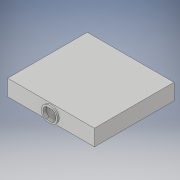
# Autodesk Inventor part: room with 15 cubicals
Saved by Autodesk Inventor 2017 (Build 210142000, 142)
## iProperties
Created: 2018-03-22
Part Number: room with 15 cubicals
Material: Generic
Document SubType Name: Modeling
Designer: Braxton
Density: 1 g/cm^3
Appearance: Default
Author: Braxton
Autodesk Inventor part; units mm, degrees
ref_plane "YZ Plane" through (0, 0, 0) normal (1, 0, 0) x (0, 1, 0)
ref_plane "XZ Plane" through (0, 0, 0) normal (0, 1, 0) x (-1, 0, 0)
ref_plane "XY Plane" through (0, 0, 0) normal (0, 0, 1) x (1, 0, 0)
sketch "Sketch1" plane through (0, 0, 0) normal (0, 1, 0) x (-1, 0, 0)
  line L0 (0, 0) -> (0, -304.8)
  line L1 (0, -304.8) -> (-203.2, -304.8)
  line L2 (-203.2, -304.8) -> (-203.2, -63.5)
  line L3 (0, 0) -> (-203.2, 0)
  line L4 (-205.3167, -63.5) -> (-205.3167, -306.9167)
  line L5 (2.1167, -306.9167) -> (2.1167, 2.1167)
  line L6 (2.1167, 2.1167) -> (-203.2, 2.1167)
  line L7 (-203.2, -63.5) -> (-205.3167, -63.5)
  line L8 (-203.2, 0) -> (-205.3167, 0)
  line L9 (-205.3167, 0) -> (-205.3167, 2.1167)
  line L10 (-205.3167, 2.1167) -> (-203.2, 2.1167)
  line L11 (0, -304.8) -> (-203.2, -304.8)
  line L12 (-281.5167, -920.75) -> (-281.5167, 2.1167) construction
  line L13 (0, -306.9167) -> (-205.3167, -306.9167)
  line L14 (0, -306.9167) -> (0, -611.7167)
  line L15 (0, -611.7167) -> (-203.2, -611.7167)
  line L16 (-203.2, -611.7167) -> (-203.2, -370.4167)
  line L17 (-205.3167, -370.4167) -> (-205.3167, -613.8333)
  line L18 (2.1167, -613.8333) -> (2.1167, -306.9167)
  line L19 (-203.2, -370.4167) -> (-205.3167, -370.4167)
  line L20 (0, -611.7167) -> (-203.2, -611.7167)
  line L21 (0, -613.8333) -> (-205.3167, -613.8333)
  line L22 (0, -613.8333) -> (0, -918.6333)
  line L23 (0, -918.6333) -> (-203.2, -918.6333)
  line L24 (-203.2, -918.6333) -> (-203.2, -677.3333)
  line L25 (-205.3167, -677.3333) -> (-205.3167, -920.75)
  line L26 (2.1167, -920.75) -> (2.1167, -613.8333)
  line L27 (-203.2, -677.3333) -> (-205.3167, -677.3333)
  line L28 (0, -918.6333) -> (-203.2, -918.6333)
  line L29 (2.1167, -920.75) -> (-205.3167, -920.75)
  line L30 (-563.0333, 0) -> (-563.0333, -304.8)
  line L31 (-563.0333, -304.8) -> (-359.8333, -304.8)
  line L32 (-359.8333, -304.8) -> (-359.8333, -63.5)
  line L33 (-563.0333, 0) -> (-359.8333, 0)
  line L34 (-357.7167, -63.5) -> (-357.7167, -306.9167)
  line L35 (-565.15, -306.9167) -> (-565.15, 2.1167)
  line L36 (-565.15, 2.1167) -> (-359.8333, 2.1167)
  line L37 (-359.8333, -63.5) -> (-357.7167, -63.5)
  line L38 (-359.8333, 0) -> (-357.7167, 0)
  line L39 (-357.7167, 0) -> (-357.7167, 2.1167)
  line L40 (-357.7167, 2.1167) -> (-359.8333, 2.1167)
  line L41 (-563.0333, -304.8) -> (-359.8333, -304.8)
  line L42 (-563.0333, -306.9167) -> (-357.7167, -306.9167)
  line L43 (-563.0333, -613.8333) -> (-357.7167, -613.8333)
  line L44 (-563.0333, -611.7167) -> (-359.8333, -611.7167)
  line L45 (-563.0333, -611.7167) -> (-359.8333, -611.7167)
  line L46 (-357.7167, -370.4167) -> (-357.7167, -613.8333)
  line L47 (-359.8333, -611.7167) -> (-359.8333, -370.4167)
  line L48 (-359.8333, -370.4167) -> (-357.7167, -370.4167)
  line L49 (-563.0333, -306.9167) -> (-563.0333, -611.7167)
  line L50 (-565.15, -613.8333) -> (-565.15, -306.9167)
  line L51 (-565.15, -920.75) -> (-357.7167, -920.75)
  line L52 (-563.0333, -918.6333) -> (-359.8333, -918.6333)
  line L53 (-563.0333, -918.6333) -> (-359.8333, -918.6333)
  line L54 (-357.7167, -677.3333) -> (-357.7167, -920.75)
  line L55 (-359.8333, -918.6333) -> (-359.8333, -677.3333)
  line L56 (-359.8333, -677.3333) -> (-357.7167, -677.3333)
  line L57 (-563.0333, -613.8333) -> (-563.0333, -918.6333)
  line L58 (-565.15, -920.75) -> (-565.15, -613.8333)
  line L59 (-641.35, -920.75) -> (-641.35, 2.1167) construction
  line L60 (-1282.7, 0) -> (-1282.7, -304.8)
  line L61 (-1282.7, -304.8) -> (-1079.5, -304.8)
  line L62 (-1079.5, -304.8) -> (-1079.5, -63.5)
  line L63 (-1282.7, 0) -> (-1079.5, 0)
  line L64 (-1077.3833, -63.5) -> (-1077.3833, -306.9167)
  line L65 (-1284.8167, -306.9167) -> (-1284.8167, 2.1167)
  line L66 (-1284.8167, 2.1167) -> (-1079.5, 2.1167)
  line L67 (-1079.5, -63.5) -> (-1077.3833, -63.5)
  line L68 (-1079.5, 0) -> (-1077.3833, 0)
  line L69 (-1077.3833, 0) -> (-1077.3833, 2.1167)
  line L70 (-1077.3833, 2.1167) -> (-1079.5, 2.1167)
  line L71 (-1282.7, -304.8) -> (-1079.5, -304.8)
  line L72 (-1001.1833, -920.75) -> (-1001.1833, 2.1167) construction
  line L73 (-1282.7, -306.9167) -> (-1077.3833, -306.9167)
  line L74 (-1282.7, -613.8333) -> (-1077.3833, -613.8333)
  line L75 (-1282.7, -611.7167) -> (-1079.5, -611.7167)
  line L76 (-1282.7, -611.7167) -> (-1079.5, -611.7167)
  line L77 (-1077.3833, -370.4167) -> (-1077.3833, -613.8333)
  line L78 (-1079.5, -611.7167) -> (-1079.5, -370.4167)
  line L79 (-1079.5, -370.4167) -> (-1077.3833, -370.4167)
  line L80 (-1282.7, -306.9167) -> (-1282.7, -611.7167)
  line L81 (-1284.8167, -613.8333) -> (-1284.8167, -306.9167)
  line L82 (-1284.8167, -920.75) -> (-1077.3833, -920.75)
  line L83 (-1282.7, -918.6333) -> (-1079.5, -918.6333)
  line L84 (-1282.7, -918.6333) -> (-1079.5, -918.6333)
  line L85 (-1077.3833, -677.3333) -> (-1077.3833, -920.75)
  line L86 (-1079.5, -918.6333) -> (-1079.5, -677.3333)
  line L87 (-1079.5, -677.3333) -> (-1077.3833, -677.3333)
  line L88 (-1282.7, -613.8333) -> (-1282.7, -918.6333)
  line L89 (-1284.8167, -920.75) -> (-1284.8167, -613.8333)
  line L90 (-719.6667, 0) -> (-719.6667, -304.8)
  line L91 (-719.6667, -304.8) -> (-922.8667, -304.8)
  line L92 (-922.8667, -304.8) -> (-922.8667, -63.5)
  line L93 (-719.6667, 0) -> (-922.8667, 0)
  line L94 (-922.8667, -63.5) -> (-924.9833, -63.5)
  line L95 (-922.8667, 0) -> (-924.9833, 0)
  line L96 (-924.9833, 0) -> (-924.9833, 2.1167)
  line L97 (-924.9833, 2.1167) -> (-922.8667, 2.1167)
  line L98 (-717.55, -306.9167) -> (-717.55, 2.1167)
  line L99 (-717.55, 2.1167) -> (-922.8667, 2.1167)
  line L100 (-719.6667, -304.8) -> (-922.8667, -304.8)
  line L101 (-924.9833, -63.5) -> (-924.9833, -306.9167)
  line L102 (-719.6667, -306.9167) -> (-924.9833, -306.9167)
  line L103 (-922.8667, -370.4167) -> (-924.9833, -370.4167)
  line L104 (-719.6667, -306.9167) -> (-719.6667, -611.7167)
  line L105 (-717.55, -613.8333) -> (-717.55, -306.9167)
  line L106 (-719.6667, -611.7167) -> (-922.8667, -611.7167)
  line L107 (-719.6667, -611.7167) -> (-922.8667, -611.7167)
  line L108 (-719.6667, -613.8333) -> (-924.9833, -613.8333)
  line L109 (-924.9833, -370.4167) -> (-924.9833, -613.8333)
  line L110 (-922.8667, -611.7167) -> (-922.8667, -370.4167)
  line L111 (-922.8667, -918.6333) -> (-922.8667, -677.3333)
  line L112 (-924.9833, -677.3333) -> (-924.9833, -920.75)
  line L113 (-719.6667, -613.8333) -> (-719.6667, -918.6333)
  line L114 (-717.55, -920.75) -> (-717.55, -613.8333)
  line L115 (-719.6667, -918.6333) -> (-922.8667, -918.6333)
  line L116 (-719.6667, -918.6333) -> (-922.8667, -918.6333)
  line L117 (-717.55, -920.75) -> (-924.9833, -920.75)
  line L118 (-922.8667, -677.3333) -> (-924.9833, -677.3333)
  dimension "d4" = 304.8
  dimension "d5" = 203.2
  dimension "d7" = 63.5
  dimension "d95" = 2.1167
  dimension "d97" = 2.1167
  dimension "d98" = 2.1167
  dimension "d99" = 304.8
  dimension "d100" = 203.2
  dimension "d102" = 2.1167
  dimension "d103" = 2.1167
  dimension "d104" = 2.1167
  dimension "d106" = 304.8
  dimension "d107" = 203.2
  dimension "d109" = 2.1167
  dimension "d110" = 2.1167
  dimension "d111" = 2.1167
  dimension "d113" = 63.5
  dimension "d114" = 63.5
  dimension "d115" = 76.2
  dimension "d117" = 76.2
  constraints: 238 end point, 80 symmetric about line, 8 perpendicular, 8 vertical, 7 horizontal, 6 collinear, 4 point on line, 1 other
  measures "d4" distance of L0.end L0.start
  measures "d5" distance of L1.end L0.end
  measures "d7" distance from line of L3 L2.end
  measures "d95" distance between parallel lines of L0 L5
  measures "d97" distance between parallel lines of L1 L13
  measures "d98" distance between parallel lines of L2 L4
  measures "d99" distance of L15.start L13.start
  measures "d100" distance of L15.end L15.start
  measures "d102" distance between parallel lines of L14 L18
  measures "d103" distance between parallel lines of L15 L21
  measures "d104" distance between parallel lines of L16 L17
  measures "d106" distance of L23.start L21.start
  measures "d107" distance of L23.end L23.start
  measures "d109" distance between parallel lines of L22 L26
  measures "d110" distance between parallel lines of L23 L29
  measures "d111" distance between parallel lines of L24 L25
  measures "d113" distance between parallel lines of L13 L19
  measures "d114" distance between parallel lines of L21 L27
  measures "d115" distance between parallel lines of L25 L12
  measures "d117" distance between parallel lines of L59 L58
extrude "cubicals" add sketch "Sketch1" along normal blind 114.3
sketch "Sketch2" plane through (0, 0, 0) normal (0, -1, 0) x (1, 0, 0)
  line L0 (1310.2167, 154.5167) -> (-27.5167, 154.5167)
  line L1 (-27.5167, 154.5167) -> (-27.5167, -1073.15)
  line L2 (-27.5167, -1073.15) -> (1310.2167, -1073.15)
  line L3 (1310.2167, -1073.15) -> (1310.2167, 154.5167)
  line L4 (-2.1167, -920.75) -> (-2.1167, 2.1167) projected
  line L5 (1284.8167, 2.1167) -> (1284.8167, -920.75) projected
  line L6 (1284.8167, -920.75) -> (1077.3833, -920.75) projected
  line L7 (717.55, 2.1167) -> (924.9833, 2.1167) projected
  point P0 (0, 0)
  dimension "d118" = 152.4
  dimension "d120" = 152.4
  dimension "d128" = 25.4
  dimension "d129" = 25.4
  constraints: 8 end point, 2 parallel, 1 horizontal, 1 perpendicular
  measures "d118" distance between parallel lines of L6 L2
  measures "d120" distance between parallel lines of L0 L7
  measures "d128" distance between parallel lines of L1 L4
  measures "d129" distance between parallel lines of L3 L5
extrude "floor" add sketch "Sketch2" along normal blind 25.4
sketch "Sketch3" plane through (0, 0, 0) normal (0, 1, 0) x (1, 0, 0)
  line L0 (-27.5167, -154.5167) -> (-27.5167, 1073.15) projected
  line L1 (-27.5167, 1073.15) -> (1310.2167, 1073.15)
  line L2 (1310.2167, 1073.15) -> (1310.2167, -154.5167)
  line L3 (1310.2167, -154.5167) -> (-27.5167, -154.5167)
  line L4 (-27.5167, -154.5167) -> (-27.5167, 1073.15)
  line L5 (-2.1167, 1047.75) -> (1284.8167, 1047.75)
  line L6 (1284.8167, 1047.75) -> (1284.8167, -129.1167)
  line L7 (1284.8167, -129.1167) -> (-2.1167, -129.1167)
  line L8 (-2.1167, -129.1167) -> (-2.1167, 1047.75)
  dimension "d130" = 25.4
  dimension "d131" = 25.4
  dimension "d132" = 25.4
  dimension "d133" = 25.4
  constraints: 16 end point, 4 parallel, 2 horizontal, 2 perpendicular
  measures "d130" distance between parallel lines of L8 L0
  measures "d131" distance between parallel lines of L5 L1
  measures "d132" distance between parallel lines of L2 L6
  measures "d133" distance between parallel lines of L3 L7
extrude "walls" add sketch "Sketch3" along normal blind 197.4749
sketch "Sketch4" plane through (-27.5167, -25.4, 154.5167) normal (0, 0, 1) x (1, 0, 0)
  line L0 (1337.7333, 0) -> (0, 0) projected
  line L1 (659.8708, 194.7333) -> (618.0667, 194.7333)
  line L2 (661.4583, 197.9083) -> (661.4583, 196.3208)
  arc A0 (659.8708, 194.7333) -> (661.4583, 196.3208) centre (659.8708, 196.3208) ccw
  line L3 (668.8667, 194.7333) -> (668.8667, 197.9083) construction
  line L4 (676.275, 197.9083) -> (676.275, 196.3208)
  line L5 (661.4583, 197.9083) -> (676.275, 197.9083)
  line L6 (659.8708, 194.7333) -> (677.8625, 194.7333) construction
  arc A1 (676.275, 196.3208) -> (677.8625, 194.7333) centre (677.8625, 196.3208) ccw
  line L7 (677.8625, 194.7333) -> (719.6667, 194.7333)
  arc A2 (618.0667, 194.7333) -> (618.0667, 25.4) centre (668.8667, 110.0667) ccw
  arc A3 (726.6597, 0) -> (611.0737, 0) centre (668.8667, 110.0667) ccw
  arc A4 (719.6667, 25.4) -> (719.6667, 194.7333) centre (668.8667, 110.0667) ccw
  line L8 (618.0667, 25.4) -> (719.6667, 25.4)
  line L9 (611.0737, 0) -> (726.6597, 0)
  point P0 (668.8667, 0)
  point P1 (668.8667, 0)
  dimension "d148" = 101.6
  dimension "d149" = 25.4
  dimension "d150" = 124.3169
  dimension "d151" = 14.8167
  dimension "d152" = 98.7374
  dimension "d153" = 98.7374
  dimension "d154" = 43.3917
  dimension "d155" = 1.5875
  dimension "d156" = 1.5875
  dimension "d157" = 41.8042
  dimension "d158" = 3.175
  constraints: 18 end point, 11 point on circle, 5 centre point, 5 horizontal, 3 midpoint, 3 symmetric about line, 2 perpendicular, 1 coincident, 1 parallel, 1 tangent, 1 vertical, 1 other
  measures "d148" distance of L1.end L7.end
  measures "d149" distance between parallel lines of L8 L9
  measures "d150" radius of A3
  measures "d151" distance of L5.start L4.start
  measures "d152" radius of A2
  measures "d153" radius of A4
  measures "d154" distance from line of L1.end L2
  measures "d155" distance from line of L7.start L4
  measures "d156" radius of A1
  measures "d157" distance of L7.start L7.end
  measures "d158" distance from line of L4.start L7
extrude "connection" add sketch "Sketch4" along normal blind 25.4
sketch "Sketch5" plane through (1310.2167, -25.4, 154.5167) normal (0, 0, 1) x (1, 0, 0)
  line L0 (-675.2167, 197.9083) -> (-668.8667, 197.9083)
  line L1 (-661.4583, 197.9083) -> (-676.275, 197.9083)
  line L2 (-675.2167, 197.9083) -> (-675.2167, 196.6845)
  line L3 (-672.9701, 194.7127) -> (-668.8667, 194.7127)
  line L4 (-668.8667, 194.7127) -> (-668.8667, 197.9083) construction
  line L5 (-675.2152, 194.7333) -> (-672.0409, 197.9076) construction
  arc A0 (-672.0402, 194.7127) -> (-675.2167, 197.9083) centre (-675.2152, 194.7333) ccw construction
  arc A1 (-675.2167, 196.6845) -> (-672.9701, 194.7127) centre (-672.9701, 196.9784) ccw
  line L6 (-662.5167, 197.9083) -> (-668.8667, 197.9083)
  line L7 (-662.5167, 197.9083) -> (-662.5167, 196.6845)
  line L8 (-664.7632, 194.7127) -> (-668.8667, 194.7127)
  line L9 (-662.5182, 194.7333) -> (-665.6924, 197.9076) construction
  arc A2 (-662.5167, 197.9083) -> (-665.6931, 194.7127) centre (-662.5182, 194.7333) ccw construction
  arc A3 (-664.7632, 194.7127) -> (-662.5167, 196.6845) centre (-664.7632, 196.9784) ccw
  line L10 (-676.275, 197.9083) -> (-661.4583, 197.9083) projected
  line L11 (-676.275, 197.9083) -> (-661.4583, 197.9083)
  point P0 (-1310.2167, 25.4)
  dimension "d164" = 6.35
  dimension "d165" = 3.175
  dimension "d166" = 45
  dimension "d167" = 2.2657
  dimension "d168" = 2.2466
  constraints: 22 end point, 10 point on circle, 8 symmetric about line, 4 centre point, 4 point on line, 2 coincident, 2 horizontal, 2 midpoint, 2 perpendicular, 1 tangent, 1 vertical, 2 other
  measures "d164" distance of L4.end L0.start
  measures "d165" distance of L0.start L5.start
  measures "d166" angle of L0 L5
  measures "d167" radius of A1
  measures "d168" horizontal distance of L3.start L2.end
extrude "light connection" add sketch "Sketch5" along normal blind 25.4 separate body
sketch "Sketch6" plane through (590.55, 0, 154.5167) normal (0, 0, 1) x (1, 0, 0)
  arc A0 (0, 169.3333) -> (0, 0) centre (50.8, 84.6667) ccw projected
  circle A1 centre (50.8, 84.6667) radius 98.7375
  arc A2 (101.6, 0) -> (101.6, 169.3333) centre (50.8, 84.6667) ccw projected
  line L0 (0, 0) -> (101.6, 0)
  line L1 (41.8042, 169.3333) -> (0, 169.3333) projected
  line L2 (101.6, 169.3333) -> (59.7958, 169.3333) projected
  line L3 (0, 169.3333) -> (101.6, 169.3333)
  point P0 (-590.55, 0)
  constraints: 4 end point, 2 horizontal, 1 centre point, 1 coincident
extrude "connection cut" cut sketch "Sketch6" against normal blind 25.4 contours L1 L3 L2 A1 L0 A0 bodies 1
sketch "Sketch7" plane through (0, 197.4749, 0) normal (0, 1, 0) x (1, 0, 0)
  line L0 (-27.5167, 1073.15) -> (-27.5167, -154.5167) projected
  line L1 (693.5899, -154.5167) -> (1310.2167, -154.5167) projected
  line L2 (-27.5167, 1073.15) -> (1310.2167, 1073.15)
  line L3 (1310.2167, 1073.15) -> (1310.2167, -154.5167)
  line L4 (1310.2167, -154.5167) -> (-27.5167, -154.5167)
  line L5 (-27.5167, -154.5167) -> (-27.5167, 1073.15)
  point P0 (0, 0)
  constraints: 8 end point, 2 parallel, 1 horizontal, 1 perpendicular
extrude "Extrusion8" add sketch "Sketch7" along normal blind 25.4 bodies 1
equation "\"d95\" = d10"
equation "\"d97\" = d95"
equation "\"d98\" = d95"
equation "\"d102\" = d105"
equation "\"d103\" = d102"
equation "\"d104\" = d102"
equation "\"d109\" = d112"
equation "\"d110\" = d109"
equation "\"d111\" = d109"
equation "\"d113\" = d7"
equation "\"d114\" = d7"
equation "\"d117\" = d115"
equation "\"d118\" = d120"
equation "\"d129\" = d128"
equation "\"d131\" = d130"
equation "\"d132\" = d130"
equation "\"d133\" = d130"
equation "\"d10\" = 2.116667"
equation "\"d105\" = 2.116667"
equation "\"d112\" = 2.116667"
body "Solid1"
body "Solid2"
